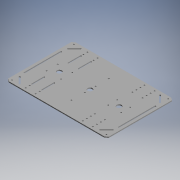
# Autodesk Inventor part: platform_board
Saved by Autodesk Inventor 2019 (Build 230136000, 136)
## iProperties
Part Number: platform_board
Material: Generic
Document SubType Name: Modeling
Designer: Jorge
Appearance: Default
Author: Jorge
Autodesk Inventor part; units mm, degrees
ref_plane "YZ Plane" through (0, 0, 0) normal (1, 0, 0) x (0, 1, 0)
ref_plane "XZ Plane" through (0, 0, 0) normal (0, 1, 0) x (-1, 0, 0)
ref_plane "XY Plane" through (0, 0, 0) normal (0, 0, 1) x (1, 0, 0)
sketch "Sketch1" plane through (0, 0, 0) normal (0, 1, 0) x (-1, 0, 0)
  line L0 (150, 100) -> (142, 100) construction
  line L1 (-150, 100) -> (-150, 94.5) construction
  line L2 (-150, -100) -> (-142, -100) construction
  line L3 (150, -100) -> (150, -94.5) construction
  line L4 (6373.4973, 0) -> (-6190.4973, 0) construction
  line L5 (0, -1054.135) -> (0, 1054.135) construction
  line L6 (142, -100) -> (150, -94.5)
  line L7 (142, 100) -> (150, 94.5)
  line L8 (150, 94.5) -> (150, 100) construction
  line L9 (142, 100) -> (-142, 100)
  line L10 (150, -94.5) -> (150, 94.5)
  line L11 (142, -100) -> (150, -100) construction
  line L12 (-150, -94.5) -> (-142, -100)
  line L13 (-142, -100) -> (142, -100)
  line L14 (-150, -94.5) -> (-150, -100) construction
  line L15 (-150, 94.5) -> (-142, 100)
  line L16 (-150, 94.5) -> (-150, -94.5)
  line L17 (-142, 100) -> (-150, 100) construction
  line L18 (150, 92) -> (-150, 92) construction
  circle A0 centre (140.5, 92) radius 2
  circle A1 centre (100, 92) radius 2
  circle A2 centre (70, 92) radius 2
  circle A3 centre (-140.5, 92) radius 2
  circle A4 centre (-100, 92) radius 2
  circle A5 centre (-70, 92) radius 2
  line L19 (0, 1054.135) -> (0, -1054.135) construction
  line L20 (150, -92) -> (-150, -92) construction
  circle A6 centre (140.5, -92) radius 2
  circle A7 centre (100, -92) radius 2
  circle A8 centre (70, -92) radius 2
  circle A9 centre (-140.5, -92) radius 2
  circle A10 centre (-100, -92) radius 2
  circle A11 centre (-70, -92) radius 2
  line L21 (-100, 100) -> (-100, 0) construction
  circle A12 centre (-100, 80) radius 2
  circle A13 centre (-100, 68) radius 2
  circle A14 centre (-100, 56) radius 2
  line L22 (-70, 100) -> (-70, 0) construction
  circle A15 centre (-70, 80) radius 2
  circle A16 centre (-70, 68) radius 2
  circle A17 centre (-70, 56) radius 2
  line L23 (-100, -100) -> (-100, 0) construction
  circle A18 centre (-100, -80) radius 2
  circle A19 centre (-100, -68) radius 2
  circle A20 centre (-100, -56) radius 2
  line L24 (-70, -100) -> (-70, 0) construction
  circle A21 centre (-70, -80) radius 2
  circle A22 centre (-70, -68) radius 2
  circle A23 centre (-70, -56) radius 2
  line L25 (70, 100) -> (70, 0) construction
  line L26 (100, 100) -> (100, 0) construction
  circle A24 centre (70, 80) radius 2
  circle A25 centre (100, 80) radius 2
  arc A26 (100, 70.5) -> (102, 72.5) centre (100, 72.5) ccw construction
  arc A27 (72, 72.5) -> (68, 72.5) centre (70, 72.5) ccw
  arc A28 (100, 38.5) -> (98, 36.5) centre (100, 36.5) ccw construction
  arc A29 (68, 36.5) -> (72, 36.5) centre (70, 36.5) ccw
  line L27 (102, 72.5) -> (102, 36.5)
  line L28 (98, 36.5) -> (98, 72.5)
  arc A30 (98, 72.5) -> (100, 70.5) centre (100, 72.5) ccw construction
  arc A31 (102, 72.5) -> (98, 72.5) centre (100, 72.5) ccw
  arc A32 (102, 36.5) -> (100, 38.5) centre (100, 36.5) ccw construction
  arc A33 (98, 36.5) -> (102, 36.5) centre (100, 36.5) ccw
  line L29 (72, 72.5) -> (72, 36.5)
  line L30 (68, 36.5) -> (68, 72.5)
  arc A34 (70, 70.5) -> (72, 72.5) centre (70, 72.5) ccw construction
  arc A35 (68, 72.5) -> (70, 70.5) centre (70, 72.5) ccw construction
  arc A36 (70, 38.5) -> (68, 36.5) centre (70, 36.5) ccw construction
  arc A37 (72, 36.5) -> (70, 38.5) centre (70, 36.5) ccw construction
  circle A38 centre (70, 16.6) radius 2
  line L31 (70, -100) -> (70, 0) construction
  line L32 (100, -100) -> (100, 0) construction
  circle A39 centre (70, -80) radius 2
  circle A40 centre (100, -80) radius 2
  arc A41 (102, -72.5) -> (100, -70.5) centre (100, -72.5) ccw construction
  arc A42 (68, -72.5) -> (72, -72.5) centre (70, -72.5) ccw
  arc A43 (98, -36.5) -> (100, -38.5) centre (100, -36.5) ccw construction
  arc A44 (72, -36.5) -> (68, -36.5) centre (70, -36.5) ccw
  line L33 (102, -72.5) -> (102, -36.5)
  line L34 (98, -36.5) -> (98, -72.5)
  arc A45 (100, -70.5) -> (98, -72.5) centre (100, -72.5) ccw construction
  arc A46 (98, -72.5) -> (102, -72.5) centre (100, -72.5) ccw
  arc A47 (100, -38.5) -> (102, -36.5) centre (100, -36.5) ccw construction
  arc A48 (102, -36.5) -> (98, -36.5) centre (100, -36.5) ccw
  line L35 (72, -72.5) -> (72, -36.5)
  line L36 (68, -36.5) -> (68, -72.5)
  arc A49 (72, -72.5) -> (70, -70.5) centre (70, -72.5) ccw construction
  arc A50 (70, -70.5) -> (68, -72.5) centre (70, -72.5) ccw construction
  arc A51 (68, -36.5) -> (70, -38.5) centre (70, -36.5) ccw construction
  arc A52 (70, -38.5) -> (72, -36.5) centre (70, -36.5) ccw construction
  circle A53 centre (70, -16.6) radius 2
  circle A54 centre (91.5, 0) radius 7
  circle A55 centre (-86.5, 0) radius 7
  circle A56 centre (0, 0) radius 7
  circle A57 centre (0, 16) radius 2
  circle A58 centre (0, -16) radius 2
  circle A59 centre (-105.8, 13.5) radius 2
  circle A60 centre (-105.8, -13.5) radius 2
  arc A61 (-138.5, 54) -> (-142.5, 54) centre (-140.5, 54) ccw
  arc A62 (-140.5, -52) -> (-142.5, -54) centre (-140.5, -54) ccw construction
  line L37 (-140.5, 54) -> (-140.5, -54) construction
  line L38 (-138.5, 54) -> (-138.5, -54)
  line L39 (-142.5, -54) -> (-142.5, 54)
  arc A63 (-140.5, 52) -> (-138.5, 54) centre (-140.5, 54) ccw construction
  arc A64 (-142.5, 54) -> (-140.5, 52) centre (-140.5, 54) ccw construction
  arc A65 (-138.5, -54) -> (-140.5, -52) centre (-140.5, -54) ccw construction
  arc A66 (-142.5, -54) -> (-138.5, -54) centre (-140.5, -54) ccw
  arc A67 (142.5, 54) -> (138.5, 54) centre (140.5, 54) ccw
  arc A68 (142.5, -54) -> (140.5, -52) centre (140.5, -54) ccw construction
  line L40 (140.5, 54) -> (140.5, -54) construction
  line L41 (138.5, 54) -> (138.5, -54)
  line L42 (142.5, -54) -> (142.5, 54)
  arc A69 (138.5, 54) -> (140.5, 52) centre (140.5, 54) ccw construction
  arc A70 (140.5, 52) -> (142.5, 54) centre (140.5, 54) ccw construction
  arc A71 (140.5, -52) -> (138.5, -54) centre (140.5, -54) ccw construction
  arc A72 (138.5, -54) -> (142.5, -54) centre (140.5, -54) ccw
  arc A73 (-117.6475, 87.8858) -> (-120.4759, 90.7142) centre (-119.0617, 89.3) ccw
  arc A74 (-136.3858, 71.9759) -> (-139.2142, 71.9759) centre (-137.8, 70.5617) ccw construction
  line L43 (-119.0617, 89.3) -> (-137.8, 70.5617) construction
  line L44 (-117.6475, 87.8858) -> (-136.3858, 69.1475)
  line L45 (-139.2142, 71.9759) -> (-120.4759, 90.7142)
  arc A75 (-120.4759, 87.8858) -> (-117.6475, 87.8858) centre (-119.0617, 89.3) ccw construction
  arc A76 (-120.4759, 90.7142) -> (-120.4759, 87.8858) centre (-119.0617, 89.3) ccw construction
  arc A77 (-136.3858, 69.1475) -> (-136.3858, 71.9759) centre (-137.8, 70.5617) ccw construction
  arc A78 (-139.2142, 71.9759) -> (-136.3858, 69.1475) centre (-137.8, 70.5617) ccw
  line L46 (-140.5, 92) -> (-119.0617, 89.3) construction
  line L47 (-140.5, 92) -> (-137.8, 70.5617) construction
  arc A79 (-120.4759, -90.7142) -> (-117.6475, -87.8858) centre (-119.0617, -89.3) ccw
  arc A80 (-139.2142, -71.9759) -> (-136.3858, -71.9759) centre (-137.8, -70.5617) ccw construction
  line L48 (-119.0617, -89.3) -> (-137.8, -70.5617) construction
  line L49 (-117.6475, -87.8858) -> (-136.3858, -69.1475)
  line L50 (-139.2142, -71.9759) -> (-120.4759, -90.7142)
  arc A81 (-117.6475, -87.8858) -> (-120.4759, -87.8858) centre (-119.0617, -89.3) ccw construction
  arc A82 (-120.4759, -87.8858) -> (-120.4759, -90.7142) centre (-119.0617, -89.3) ccw construction
  arc A83 (-136.3858, -71.9759) -> (-136.3858, -69.1475) centre (-137.8, -70.5617) ccw construction
  arc A84 (-136.3858, -69.1475) -> (-139.2142, -71.9759) centre (-137.8, -70.5617) ccw
  line L51 (-140.5, -92) -> (-137.8, -70.5617) construction
  arc A85 (117.6475, 92) -> (120.4759, 92) centre (119.0617, 90.5858) ccw construction
  arc A86 (136.3858, 70.4332) -> (139.2142, 73.2617) centre (137.8, 71.8475) ccw
  line L52 (119.0617, 90.5858) -> (137.8, 71.8475) construction
  line L53 (117.6475, 89.1716) -> (136.3858, 70.4332)
  line L54 (139.2142, 73.2617) -> (120.4759, 92)
  arc A87 (117.6475, 89.1716) -> (117.6475, 92) centre (119.0617, 90.5858) ccw construction
  arc A88 (120.4759, 92) -> (117.6475, 89.1716) centre (119.0617, 90.5858) ccw
  arc A89 (139.2142, 70.4332) -> (136.3858, 70.4332) centre (137.8, 71.8475) ccw construction
  arc A90 (139.2142, 73.2617) -> (139.2142, 70.4332) centre (137.8, 71.8475) ccw construction
  line L55 (150, -92) -> (-150, -92) construction
  arc A91 (120.4759, -92) -> (117.6475, -92) centre (119.0617, -90.5858) ccw construction
  arc A92 (139.2142, -73.2617) -> (136.3858, -70.4332) centre (137.8, -71.8475) ccw
  line L56 (119.0617, -90.5858) -> (137.8, -71.8475) construction
  line L57 (117.6475, -89.1716) -> (136.3858, -70.4332)
  line L58 (139.2142, -73.2617) -> (120.4759, -92)
  arc A93 (117.6475, -92) -> (117.6475, -89.1716) centre (119.0617, -90.5858) ccw construction
  arc A94 (117.6475, -89.1716) -> (120.4759, -92) centre (119.0617, -90.5858) ccw
  arc A95 (136.3858, -70.4332) -> (139.2142, -70.4332) centre (137.8, -71.8475) ccw construction
  arc A96 (139.2142, -70.4332) -> (139.2142, -73.2617) centre (137.8, -71.8475) ccw construction
  line L59 (-86.5, 23.4128) -> (-86.5, -26.7268) construction
  line L60 (-6546.4973, 0) -> (6017.4973, 0) construction
  circle A97 centre (-67.2, 13.5) radius 2
  circle A98 centre (-67.2, -13.5) radius 2
  line L61 (91.5, 21.1732) -> (91.5, -21.9498) construction
  line L62 (-6190.4973, 0) -> (6373.4973, 0) construction
  line L63 (113, 100) -> (113, 0) construction
  circle A99 centre (113, 16.6) radius 2
  line L64 (113, -100) -> (113, 0) construction
  circle A100 centre (113, -16.6) radius 2
  line L65 (6729.4973, 0) -> (-5834.4973, 0) construction
  circle A101 centre (0, 55.5) radius 2
  circle A102 centre (0, -55.5) radius 2
  dimension "d0" = 300
  dimension "d1" = 200
  dimension "d2" = 8
  dimension "d3" = 5.5
  dimension "d4" = 5.5
  dimension "d5" = 8
  dimension "d6" = 8
  dimension "d7" = 5.5
  dimension "d8" = 5.5
  dimension "d9" = 8
  dimension "d10" = 8
  dimension "d11" = 4
  dimension "d12" = 4
  dimension "d13" = 4
  dimension "d14" = 9.5
  dimension "d15" = 50
  dimension "d16" = 80
  dimension "d17" = 4
  dimension "d18" = 4
  dimension "d19" = 4
  dimension "d20" = 9.5
  dimension "d21" = 50
  dimension "d22" = 80
  dimension "d23" = 4
  dimension "d24" = 4
  dimension "d25" = 4
  dimension "d26" = 44
  dimension "d27" = 32
  dimension "d28" = 20
  dimension "d29" = 4
  dimension "d30" = 4
  dimension "d31" = 4
  dimension "d32" = 20
  dimension "d33" = 32
  dimension "d34" = 44
  dimension "d35" = 4
  dimension "d36" = 4
  dimension "d37" = 20
  dimension "d38" = 20
  dimension "d39" = 4
  dimension "d40" = 4
  dimension "d41" = 7.5
  dimension "d42" = 7.5
  dimension "d43" = 4
  dimension "d44" = 36
  dimension "d45" = 4
  dimension "d46" = 36
  dimension "d47" = 4
  dimension "d48" = 16.6
  dimension "d49" = 14
  dimension "d50" = 14
  dimension "d51" = 58.5
  dimension "d52" = 63.5
  dimension "d53" = 14
  dimension "d54" = 4
  dimension "d55" = 16
  dimension "d56" = 4
  dimension "d57" = 13.5
  dimension "d58" = 44.2
  dimension "d59" = 4
  dimension "d60" = 4
  dimension "d61" = 9.5
  dimension "d62" = 108
  dimension "d63" = 4
  constraints: 124 end point, 120 point on circle, 103 centre point, 63 point on line, 58 vertical alignment, 41 equal radius, 24 tangent, 22 parallel, 22 symmetric about line, 9 perpendicular, 9 vertical, 4 horizontal, 1 coincident, 1 equal length, 41 other
  measures "d0" distance of L3.start L2.start
  measures "d1" distance of L2.start L1.start
  measures "d2" distance of L3.start L6.start
  measures "d3" distance of L3.start L3.end
  measures "d4" distance of L0.start L7.end
  measures "d5" distance of L0.start L0.end
  measures "d6" distance of L2.end L2.start
  measures "d7" distance of L2.start L12.start
  measures "d8" distance of L1.start L1.end
  measures "d9" distance of L9.end L1.start
  measures "d11" diameter of A0
  measures "d12" diameter of A1
  measures "d13" diameter of A2
  measures "d14" distance from line of L10 A0.centre
  measures "d15" distance from line of L10 A1.centre
  measures "d16" distance from line of L10 A2.centre
  measures "d17" diameter of A3
  measures "d18" diameter of A4
  measures "d19" diameter of A5
  measures "d20" distance from line of L16 L46.start
  measures "d21" distance from line of L16 A4.centre
  measures "d22" distance from line of L16 A5.centre
  measures "d23" diameter of A12
  measures "d24" diameter of A13
  measures "d25" diameter of A14
  measures "d26" distance from line of L9 A14.centre
  measures "d27" distance from line of L9 A13.centre
  measures "d28" distance from line of L9 A12.centre
  measures "d29" diameter of A15
  measures "d30" diameter of A16
  measures "d31" diameter of A17
  measures "d32" distance from line of L9 A15.centre
  measures "d33" distance from line of L9 A16.centre
  measures "d34" distance from line of L9 A17.centre
  measures "d35" diameter of A24
  measures "d36" diameter of A25
  measures "d37" distance from line of L9 A25.centre
  measures "d38" distance from line of L9 A24.centre
  measures "d39" diameter of A26
  measures "d40" diameter of A27
  measures "d41" distance of A26.centre A25.centre
  measures "d42" distance of A24.centre A27.centre
  measures "d43" diameter of A28
  measures "d44" distance of A28.centre A26.centre
  measures "d45" diameter of A29
  measures "d46" distance of A29.centre A27.centre
  measures "d47" diameter of A38
  measures "d49" diameter of A54
  measures "d50" diameter of A55
  measures "d51" distance from line of L10 A54.centre
  measures "d52" distance from line of L16 A55.centre
  measures "d53" diameter of A56
  measures "d54" diameter of A57
  measures "d55" distance of A56.centre A57.centre
  measures "d56" diameter of A59
  measures "d58" distance from line of L16 A59.centre
  measures "d59" diameter of A61
  measures "d60" diameter of A62
  measures "d61" distance between parallel lines of L16 L37
  measures "d62" distance of L37.end L37.start
  measures "d63" diameter of A73
extrude "Extrusion2" add sketch "Sketch1" along normal blind 3
body "Solid2"
